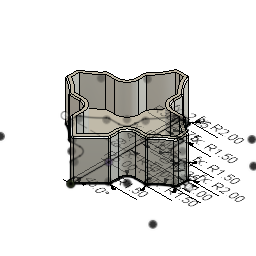
Faztek_cap v27 (Autodesk Fusion 360 design; units mm, degrees)
Autodesk Fusion 360 part; units mm, degrees
sketch "Sketch2" plane through (0, 0, 0) normal (0, 1, 0) x (1, 0, 0)
  line L0 (-0.2059, -23.3189) -> (11.4298, -11.6832)
  line L1 (11.8691, -10.6225) -> (11.8691, -5.6689)
  line L2 (16.8691, -0.6689) -> (22.9441, -0.6689)
  line L3 (34.1441, 8.7311) -> (34.1441, 14.0311)
  line L4 (22.9441, 23.4311) -> (16.8691, 23.4311)
  line L5 (11.8691, 28.4311) -> (11.8691, 33.3848)
  line L6 (2.4441, 46.0811) -> (-0.2059, 46.0811)
  line L7 (-0.2059, 46.0811) -> (-0.2059, -23.3189)
  arc A0 (16.8691, -0.6689) -> (11.8691, -5.6689) centre (16.8691, -5.6689) ccw
  arc A1 (11.8691, 28.4311) -> (16.8691, 23.4311) centre (16.8691, 28.4311) ccw
  arc A2 (33.0624, 6.9544) -> (24.0819, -0.1464) centre (46.8372, -19.6962) ccw
  arc A3 (24.0819, 22.9086) -> (33.0624, 15.8078) centre (46.8372, 42.4585) ccw
  arc A4 (4.294, 44.8412) -> (11.4012, 34.4733) centre (32.0429, 56.243) ccw
  arc A5 (11.4298, -11.6832) -> (11.8691, -10.6225) centre (10.3691, -10.6225) ccw
  arc A6 (22.9441, -0.6689) -> (24.0819, -0.1464) centre (22.9441, 0.8311) ccw
  arc A7 (33.0624, 6.9544) -> (34.1441, 8.7311) centre (32.1441, 8.7311) ccw
  arc A8 (34.1441, 14.0311) -> (33.0624, 15.8078) centre (32.1441, 14.0311) ccw
  arc A9 (24.0819, 22.9086) -> (22.9441, 23.4311) centre (22.9441, 21.9311) ccw
  arc A10 (11.8691, 33.3848) -> (11.4012, 34.4733) centre (10.3691, 33.3848) ccw
  arc A11 (4.294, 44.8412) -> (2.4441, 46.0811) centre (2.4441, 44.0811) ccw
  line L8 (-34.5559, 8.7311) -> (-34.5559, 14.0311)
  arc A12 (-24.4937, -0.1464) -> (-33.4742, 6.9544) centre (-47.249, -19.6962) ccw
  arc A13 (-23.3559, 23.4311) -> (-24.4937, 22.9086) centre (-23.3559, 21.9311) ccw
  arc A14 (-11.813, 34.4733) -> (-12.2809, 33.3848) centre (-10.7809, 33.3848) ccw
  arc A15 (-11.813, 34.4733) -> (-4.7058, 44.8412) centre (-32.4547, 56.243) ccw
  line L9 (-12.2809, -10.6225) -> (-12.2809, -5.6689)
  arc A16 (-33.4742, 15.8078) -> (-24.4937, 22.9086) centre (-47.249, 42.4585) ccw
  arc A17 (-2.8559, 46.0811) -> (-4.7058, 44.8412) centre (-2.8559, 44.0811) ccw
  arc A18 (-24.4937, -0.1464) -> (-23.3559, -0.6689) centre (-23.3559, 0.8311) ccw
  line L10 (-0.2059, -23.3189) -> (-11.8416, -11.6832)
  arc A19 (-34.5559, 8.7311) -> (-33.4742, 6.9544) centre (-32.5559, 8.7311) ccw
  arc A20 (-12.2809, -5.6689) -> (-17.2809, -0.6689) centre (-17.2809, -5.6689) ccw
  line L11 (-17.2809, -0.6689) -> (-23.3559, -0.6689)
  line L12 (-2.8559, 46.0811) -> (-0.2059, 46.0811)
  arc A21 (-33.4742, 15.8078) -> (-34.5559, 14.0311) centre (-32.5559, 14.0311) ccw
  arc A22 (-12.2809, -10.6225) -> (-11.8416, -11.6832) centre (-10.7809, -10.6225) ccw
  line L13 (-12.2809, 28.4311) -> (-12.2809, 33.3848)
  arc A23 (-17.2809, 23.4311) -> (-12.2809, 28.4311) centre (-17.2809, 28.4311) ccw
  line L14 (-23.3559, 23.4311) -> (-17.2809, 23.4311)
  line L15 (-38.524, 11.3811) -> (38.1122, 11.3811) construction
  line L16 (22.9441, -0.6689) -> (22.9441, 23.4311) construction
  point P0 (-0.4118, 0)
  dimension "d1" = 5
  dimension "d2" = 30
  dimension "d3" = 30
  dimension "d4" = 30
  dimension "d5" = 1.5
  dimension "d8" = 69.4
  dimension "d9" = 12.075
  dimension "d10" = 34.35
  dimension "d11" = 24.1
  dimension "d34" = 23.15
  dimension "d36" = 5.3
  dimension "d37" = 2.65
  dimension "d38" = 5
  dimension "d39" = 1.5
  dimension "d40" = 2
  dimension "d41" = 2
  dimension "d42" = 1.5
  dimension "d43" = 1.5
  dimension "d44" = 2
  dimension "d46" = 45
  constraint vertical L1
  constraint perpendicular L1 L2
  constraint vertical L3
  constraint horizontal L4
  constraint perpendicular L4 L5
  constraint perpendicular L5 L6
  constraint perpendicular L6 L7
  constraint tangent L2 A0
  constraint tangent L1 A0
  constraint tangent L4 A1
  constraint tangent L5 A1
  constraint tangent L0 A5
  constraint tangent L1 A5
  constraint tangent L2 A6
  constraint tangent A2 A6
  constraint tangent L3 A7
  constraint tangent A2 A7
  constraint tangent L3 A8
  constraint tangent A3 A8
  constraint tangent L4 A9
  constraint tangent A3 A9
  constraint tangent L5 A10
  constraint tangent A4 A10
  constraint tangent L6 A11
  constraint tangent A4 A11
  constraint symmetric origin L7 P0
  constraint symmetric L0.start L7 L10.start
  constraint symmetric L6.end L7 L12.end
  constraint symmetric L7 L2.start A20.end
  constraint symmetric L7 L1.end L9.end
  constraint symmetric L7 A0 A20
  constraint symmetric L7 L4.end A23.start
  constraint symmetric L7 L5.start L13.start
  constraint symmetric L7 A1 A23
  constraint symmetric L7 A2 A12
  constraint symmetric L7 A3 A16
  constraint symmetric L7 A4 A15
  constraint symmetric L7 L0.end L10.end
  constraint symmetric L7 L1.start L9.start
  constraint symmetric L7 A5 A22
  constraint symmetric L7 L2.end A18.end
  constraint symmetric L7 A2.end A12.start
  constraint symmetric L7 A6 A18
  constraint symmetric L7 L3.start L8.start
  constraint symmetric L7 A2.start A12.end
  constraint symmetric L7 A7 A19
  constraint symmetric L7 L3.end L8.end
  constraint symmetric L7 A3.end A16.start
  constraint symmetric L7 A8 A21
  constraint symmetric L7 L4.start A13.start
  constraint symmetric L7 A3.start A13.end
  constraint symmetric L7 A9 A13
  constraint symmetric L7 L5.end A14.end
  constraint symmetric L7 A4.end A14.start
  constraint symmetric L7 A10 A14
  constraint symmetric L7 L6.start A17.start
  constraint symmetric L7 A4.start A15.end
  constraint symmetric L7 A11 A17
  constraint horizontal L15
  constraint midpoint L7 L15
  constraint symmetric L2 L4 L15
  constraint symmetric L3.start L3.end L15
  constraint parallel L7 L16
  constraint collinear L1 L5
  constraint symmetric L1.start L5.end L15
  measures "d1" radius of A0
  measures "d2" radius of A4
  measures "d3" radius of A3
  measures "d4" radius of A2
  measures "d5" radius of A5
  measures "d8" distance of L0.start L6.end
  measures "d9" distance of L5 L7
  measures "d10" distance of L3 L7
  measures "d11" distance of L2 L4
  measures "d34" distance of L7 L4.start
  measures "d36" distance of L3.start L3.end
  measures "d37" distance of L6.end L6.start
  measures "d38" radius of A1
  measures "d39" radius of A6
  measures "d40" radius of A7
  measures "d41" radius of A8
  measures "d42" radius of A9
  measures "d43" radius of A10
  measures "d44" radius of A11
  measures "d46" angle of L0 L7
extrude "Extrude1" add sketch "Sketch2" along normal blind 25
shell "Shell1" thickness 2.4 removed faces 1 at (4.2262, 25, -15.973)
fillet "Fillet1" radius 1 1 edges at (-0.2059, 12.5, 23.3189)
chamfer "Chamfer1" distance 0.7 angle 45 39 edges at (-12.1667, 25, 11.1966) (-6.3773, 25, 17.1475) (-0.2059, 25, 22.9047) (5.9655, 25, 17.1475) (11.7549, 25, 11.1966) (11.8691, 25, 8.1457) (13.3336, 25, 2.1333) (19.9066, 25, 0.6689) (23.5701, 25, 0.532) (28.2303, 25, -3.8364) (33.8524, 25, -7.6911) (34.1441, 25, -11.3811) (33.8524, 25, -15.0712) (28.2303, 25, -18.9259) (23.5701, 25, -23.2943) (19.9066, 25, -23.4311) (13.3336, 25, -24.8956) (11.8691, 25, -30.908) (11.7472, 25, -33.9772) (7.2985, 25, -39.2809) (3.5576, 25, -45.7425) (1.1191, 25, -46.0811) (-1.5309, 25, -46.0811) (-3.9694, 25, -45.7425) (-7.7103, 25, -39.2809) (-12.159, 25, -33.9772) (-12.2809, 25, -30.908) (-13.7454, 25, -24.8956) (-20.3184, 25, -23.4311) (-23.9819, 25, -23.2943) (-28.6421, 25, -18.9259) (-34.2642, 25, -15.0712) (-34.5559, 25, -11.3811) (-34.2642, 25, -7.6911) (-28.6421, 25, -3.8364) (-23.9819, 25, 0.532) (-20.3184, 25, 0.6689) (-13.7454, 25, 2.1333) (-12.2809, 25, 8.1457)
chamfer "Chamfer2" distance 0.7 angle 45 39 edges at (-34.2642, 0, -7.6911) (-34.5559, 0, -11.3811) (-34.2642, 0, -15.0712) (-28.6421, 0, -18.9259) (-23.9819, 0, -23.2943) (-20.3184, 0, -23.4311) (-13.7454, 0, -24.8956) (-12.2809, 0, -30.908) (-12.159, 0, -33.9772) (-7.7103, 0, -39.2809) (-3.9694, 0, -45.7425) (-1.5309, 0, -46.0811) (1.1191, 0, -46.0811) (3.5576, 0, -45.7425) (7.2985, 0, -39.2809) (11.7472, 0, -33.9772) (11.8691, 0, -30.908) (13.3336, 0, -24.8956) (19.9066, 0, -23.4311) (23.5701, 0, -23.2943) (28.2303, 0, -18.9259) (33.8524, 0, -15.0712) (34.1441, 0, -11.3811) (33.8524, 0, -7.6911) (28.2303, 0, -3.8364) (23.5701, 0, 0.532) (19.9066, 0, 0.6689) (13.3336, 0, 2.1333) (11.8691, 0, 8.1457) (11.7549, 0, 11.1966) (5.9655, 0, 17.1475) (-0.2059, 0, 22.9047) (-6.3773, 0, 17.1475) (-12.1667, 0, 11.1966) (-12.2809, 0, 8.1457) (-13.7454, 0, 2.1333) (-20.3184, 0, 0.6689) (-23.9819, 0, 0.532) (-28.6421, 0, -3.8364)
extrude "Extrude5" add 1 faces at (3.6216, 2.4, -15.4491) along direction (0, 1, 0) blind 4
equation "d3 = d2"
equation "d4 = d2"
equation "d8 = 69.8 mm - 0.4 mm"
equation "d9 = ( 24.35 / 2 ) * 1 mm - 0.1 mm"
equation "d10 = ( 69.1 / 2 ) * 1 mm - 0.2 mm"
equation "d11 = 24.5 mm - 0.4 mm"
equation "d34 = ( 46.7 / 2 ) * 1 mm - 0.2 mm"
equation "d37 = d36 / 2"
equation "d38 = d1"
equation "d39 = d5"
equation "d41 = d40"
equation "d42 = d5"
equation "d43 = d5"
equation "d44 = d40"
named bodies: "EdgeBody"
